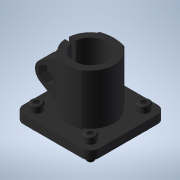
# Autodesk Inventor part: BZA-GP
Saved by Autodesk Inventor 2021 (Build 250183000, 183)
## iProperties
Created: 2025-06-23
Part Number: BZA-GP
Material: Generic
Catalog Web Link: www.cadenas.de
Description: Stands-Accessories
Vendor: RNA
Document SubType Name: Modeling
Designer: psAdmin
Manufacturer: RNA
Mass: 155.079 g
Surface Area: 462.762 cm^2
Volume: 155.079 cm^3
Density: 1 g/cm^3
Appearance: PSOLRGB-175-175-175
Category: PARTsolutions
Company: RNA
Title: BZA-GP
Author: Cadenas PARTsolutions
Comments: Accessories
PSOL_IDENT_0: {$CADENAS_DATA/23d-libs/rna/bunker/zubehoer/parts/bza_grund_110.prj},152 {VTYP=3D},{NB=BZA-GP},{LINA=
PSOL_IDENT_1: BZA-GP},{NN=Stands},{DATE=06.06.2017 07:14:33},{GEOMDATE=27.04.2017 12:08:00},{VERSION=},{LINEID=10}
PSOL_IDENT_2: ,{WBVAR=},{WBNUMERIC=}  {NB=BZA-GP},{LINA=BZA-GP},{KT=DUMMY},{IDNR=BZA-GP}
NB: BZA-GP
NN: Stands
NT: Accessories
NBSYN: $IDNR.
LINA: BZA-GP
CATALOG: Rhein-Nadel-Automation
IDNR: BZA-GP
SUPPLIER: RNA
ARTICLENO: BZA-GP
BOMINFO: BZA-GP
CREATOR: CADENAS GmbH
Autodesk Inventor part; units mm, degrees
ref_plane "YZ Plane" through (0, 0, 0) normal (1, 0, 0) x (0, 1, 0)
ref_plane "XZ Plane" through (0, 0, 0) normal (0, 1, 0) x (-1, 0, 0)
ref_plane "XY Plane" through (0, 0, 0) normal (0, 0, 1) x (1, 0, 0)
sketch "Sketch_1" plane through (0, 0, 0) normal (0, 1, 0) x (-1, 0, 0)
  line L0 (45, 2.5) -> (45, 35)
  arc A0 (45, 35) -> (35, 45) centre (35, 35) ccw
  line L1 (35, 45) -> (-35, 45)
  arc A1 (-35, 45) -> (-45, 35) centre (-35, 35) ccw
  line L2 (-45, 35) -> (-45, -35)
  arc A2 (-45, -35) -> (-35, -45) centre (-35, -35) ccw
  line L3 (-35, -45) -> (35, -45)
  arc A3 (35, -45) -> (45, -35) centre (35, -35) ccw
  line L4 (45, -35) -> (45, -2.5)
  line L5 (45, -2.5) -> (0, -2.5)
  line L6 (0, -2.5) -> (0, 2.5)
  line L7 (0, 2.5) -> (45, 2.5)
  arc A4 (-26.9948, -33.0052) -> (-33.0052, -26.9948) centre (-30, -30) ccw
  line L8 (-33.0052, -26.9948) -> (-35.0052, -28.9948)
  arc A5 (-35.0052, -28.9948) -> (-28.9948, -35.0052) centre (-32, -32) ccw
  line L9 (-28.9948, -35.0052) -> (-26.9948, -33.0052)
  arc A6 (-33.0052, 26.9948) -> (-26.9948, 33.0052) centre (-30, 30) ccw
  line L10 (-26.9948, 33.0052) -> (-28.9948, 35.0052)
  arc A7 (-28.9948, 35.0052) -> (-35.0052, 28.9948) centre (-32, 32) ccw
  line L11 (-35.0052, 28.9948) -> (-33.0052, 26.9948)
  arc A8 (28.9948, -35.0052) -> (35.0052, -28.9948) centre (32, -32) ccw
  line L12 (35.0052, -28.9948) -> (33.0052, -26.9948)
  arc A9 (33.0052, -26.9948) -> (26.9948, -33.0052) centre (30, -30) ccw
  line L13 (26.9948, -33.0052) -> (28.9948, -35.0052)
  arc A10 (35.0052, 28.9948) -> (28.9948, 35.0052) centre (32, 32) ccw
  line L14 (28.9948, 35.0052) -> (26.9948, 33.0052)
  arc A11 (26.9948, 33.0052) -> (33.0052, 26.9948) centre (30, 30) ccw
  line L15 (33.0052, 26.9948) -> (35.0052, 28.9948)
  constraints: 32 end point, 24 point on circle, 12 centre point
extrude "Extrusion1" add sketch "Sketch_1" along normal blind 10
sketch "Sketch_2" plane through (0, 10, 0) normal (0, 1, 0) x (1, 0, 0)
  arc A0 (-27.8882, -2.5) -> (-15, -23.6432) centre (0, 0) ccw
  line L0 (-15, -23.6432) -> (-15, -25.4856)
  arc A1 (-15, -25.4856) -> (15, -25.4856) centre (0, 18) ccw
  line L1 (15, -25.4856) -> (15, -23.6432)
  arc A2 (15, -23.6432) -> (15, 23.6432) centre (0, 0) ccw
  line L2 (15, 23.6432) -> (15, 25.4856)
  arc A3 (15, 25.4856) -> (-15, 25.4856) centre (0, -18) ccw
  line L3 (-15, 25.4856) -> (-15, 23.6432)
  arc A4 (-15, 23.6432) -> (-27.8882, 2.5) centre (0, 0) ccw
  line L4 (-27.8882, 2.5) -> (0, 2.5)
  line L5 (0, 2.5) -> (0, -2.5)
  line L6 (0, -2.5) -> (-27.8882, -2.5)
  constraints: 14 end point, 10 point on circle, 5 centre point
extrude "Extrusion2" add sketch "Sketch_2" along normal blind 60
sketch "Sketch_3" plane through (0, 0, 0) normal (1, 0, 0) x (0, 1, 0)
  line L0 (40, -36.5) -> (40, -26.5)
  line L1 (40, -26.5) -> (47.5, -26.5)
  line L2 (47.5, -26.5) -> (47.5, -36.5)
  line L3 (47.5, -36.5) -> (40, -36.5)
  line L4 (40, -36.5) -> (40, -26.5)
  constraints: 10 end point
revolve "Revolution1" cut sketch "Sketch_3" angle 360 about axis through (0, 40, -36.5) along (0, 0, -1)
sketch "Sketch_4" plane through (0, 0, 2.5) normal (0, 0, 1) x (1, 0, 0)
  arc A0 (-39.6142, 51.1916) -> (-39.6142, 28.8084) centre (-33, 40) ccw
  line L0 (-39.6142, 28.8084) -> (-19.1, 16.6845)
  line L1 (-19.1, 16.6845) -> (-19.1, 63.3155)
  line L2 (-19.1, 63.3155) -> (-39.6142, 51.1916)
  constraints: 6 end point, 2 point on circle, 1 centre point
extrude "Extrusion3" add sketch "Sketch_4" along normal blind 17.5
sketch "Sketch_5" plane through (0, 0, -2.5) normal (0, 0, 1) x (1, 0, 0)
  arc A0 (-39.6142, 51.1916) -> (-39.6142, 28.8084) centre (-33, 40) ccw
  line L0 (-39.6142, 28.8084) -> (-19.1, 16.6845)
  line L1 (-19.1, 16.6845) -> (-19.1, 63.3155)
  line L2 (-19.1, 63.3155) -> (-39.6142, 51.1916)
  constraints: 6 end point, 2 point on circle, 1 centre point
extrude "Extrusion4" add sketch "Sketch_5" against normal blind 17.5
sketch "Sketch_6" plane through (0, 0, 0) normal (0, 1, 0) x (-1, 0, 0)
  circle A0 centre (0, 0) radius 20.085
  constraints: 1 centre point
extrude "Extrusion5" cut sketch "Sketch_6" along normal blind 70
sketch "Sketch_7" plane through (0, 0, 20) normal (0, 0, 1) x (1, 0, 0)
  line L0 (-41.5, 35.0925) -> (-33, 30.185)
  line L1 (-33, 30.185) -> (-24.5, 35.0925)
  line L2 (-24.5, 35.0925) -> (-24.5, 44.9075)
  line L3 (-24.5, 44.9075) -> (-33, 49.815)
  line L4 (-33, 49.815) -> (-41.5, 44.9075)
  line L5 (-41.5, 44.9075) -> (-41.5, 35.0925)
  constraints: 12 end point
extrude "Extrusion6" cut sketch "Sketch_7" against normal blind 10
sketch "Sketch_8" plane through (0, 0, -20) normal (0, 0, 1) x (1, 0, 0)
  line L0 (-41.5, 35.0925) -> (-33, 30.185)
  line L1 (-33, 30.185) -> (-24.5, 35.0925)
  line L2 (-24.5, 35.0925) -> (-24.5, 44.9075)
  line L3 (-24.5, 44.9075) -> (-33, 49.815)
  line L4 (-33, 49.815) -> (-41.5, 44.9075)
  line L5 (-41.5, 44.9075) -> (-41.5, 35.0925)
  constraints: 12 end point
extrude "Extrusion7" cut sketch "Sketch_8" along normal blind 10
sketch "Sketch_10" plane through (0, 0, 0) normal (0, 0, 1) x (1, 0, 0)
  circle A0 centre (-33, 40) radius 5.25
  constraints: 1 centre point
extrude "Extrusion8" cut sketch "Sketch_10" along normal mid plane 60
sketch "Sketch_12" plane through (0, 0, 32) normal (0, 0, 1) x (1, 0, 0)
  line L0 (32, -10) -> (32, 18)
  line L1 (32, 18) -> (37.7, 18)
  line L2 (37.7, 18) -> (38.5, 17.2)
  line L3 (38.5, 17.2) -> (38.5, 10.34)
  line L4 (38.5, 10.34) -> (38.16, 10)
  line L5 (38.16, 10) -> (36.8083, 10)
  arc A0 (36.8083, 10) -> (36.4619, 9.8) centre (36.8083, 9.6) ccw
  line L6 (36.4619, 9.8) -> (36.0536, 9.0928)
  arc A1 (36.0536, 9.0928) -> (36, 8.8928) centre (36.4, 8.8928) ccw
  line L7 (36, 8.8928) -> (36, -9.233)
  line L8 (36, -9.233) -> (35.233, -10)
  line L9 (35.233, -10) -> (32, -10)
  line L10 (32, -10) -> (32, 18)
  constraints: 22 end point, 4 point on circle, 2 centre point
revolve "Revolution2" add sketch "Sketch_12" angle 360 about axis through (32, -10, 32) along (0, -1, 0)
thread "Thread1" size "M8x1.25" class "6g" standard "ISO Metric profile" length 17.233
sketch "Sketch_13" plane through (32, 18, 32) normal (0, 1, 0) x (1, 0, 0)
  line L0 (-3, -1.7321) -> (0, -3.4641)
  line L1 (0, -3.4641) -> (3, -1.7321)
  line L2 (3, -1.7321) -> (3, 1.7321)
  line L3 (3, 1.7321) -> (0, 3.4641)
  line L4 (0, 3.4641) -> (-3, 1.7321)
  line L5 (-3, 1.7321) -> (-3, -1.7321)
  constraints: 12 end point
extrude "Extrusion9" cut sketch "Sketch_13" against normal blind 4
sketch "Sketch_14" plane through (0, 0, 32) normal (0, 0, 1) x (1, 0, 0)
  line L0 (-32, -10) -> (-32, 18)
  line L1 (-32, 18) -> (-26.3, 18)
  line L2 (-26.3, 18) -> (-25.5, 17.2)
  line L3 (-25.5, 17.2) -> (-25.5, 10.34)
  line L4 (-25.5, 10.34) -> (-25.84, 10)
  line L5 (-25.84, 10) -> (-27.1917, 10)
  arc A0 (-27.1917, 10) -> (-27.5381, 9.8) centre (-27.1917, 9.6) ccw
  line L6 (-27.5381, 9.8) -> (-27.9464, 9.0928)
  arc A1 (-27.9464, 9.0928) -> (-28, 8.8928) centre (-27.6, 8.8928) ccw
  line L7 (-28, 8.8928) -> (-28, -9.233)
  line L8 (-28, -9.233) -> (-28.767, -10)
  line L9 (-28.767, -10) -> (-32, -10)
  line L10 (-32, -10) -> (-32, 18)
  constraints: 22 end point, 4 point on circle, 2 centre point
revolve "Revolution3" add sketch "Sketch_14" angle 360 about axis through (-32, -10, 32) along (0, -1, 0)
thread "Thread2" size "M8x1.25" class "6g" standard "ISO Metric profile" length 17.233
sketch "Sketch_15" plane through (-32, 18, 32) normal (0, 1, 0) x (1, 0, 0)
  line L0 (-3, -1.7321) -> (0, -3.4641)
  line L1 (0, -3.4641) -> (3, -1.7321)
  line L2 (3, -1.7321) -> (3, 1.7321)
  line L3 (3, 1.7321) -> (0, 3.4641)
  line L4 (0, 3.4641) -> (-3, 1.7321)
  line L5 (-3, 1.7321) -> (-3, -1.7321)
  constraints: 12 end point
extrude "Extrusion10" cut sketch "Sketch_15" against normal blind 4
sketch "Sketch_16" plane through (0, 0, -32) normal (0, 0, 1) x (1, 0, 0)
  line L0 (32, -10) -> (32, 18)
  line L1 (32, 18) -> (37.7, 18)
  line L2 (37.7, 18) -> (38.5, 17.2)
  line L3 (38.5, 17.2) -> (38.5, 10.34)
  line L4 (38.5, 10.34) -> (38.16, 10)
  line L5 (38.16, 10) -> (36.8083, 10)
  arc A0 (36.8083, 10) -> (36.4619, 9.8) centre (36.8083, 9.6) ccw
  line L6 (36.4619, 9.8) -> (36.0536, 9.0928)
  arc A1 (36.0536, 9.0928) -> (36, 8.8928) centre (36.4, 8.8928) ccw
  line L7 (36, 8.8928) -> (36, -9.233)
  line L8 (36, -9.233) -> (35.233, -10)
  line L9 (35.233, -10) -> (32, -10)
  line L10 (32, -10) -> (32, 18)
  constraints: 22 end point, 4 point on circle, 2 centre point
revolve "Revolution4" add sketch "Sketch_16" angle 360 about axis through (32, -10, -32) along (0, -1, 0)
thread "Thread3" size "M8x1.25" class "6g" standard "ISO Metric profile" length 17.233
sketch "Sketch_17" plane through (0, 0, -32) normal (0, 0, 1) x (1, 0, 0)
  line L0 (-32, -10) -> (-32, 18)
  line L1 (-32, 18) -> (-26.3, 18)
  line L2 (-26.3, 18) -> (-25.5, 17.2)
  line L3 (-25.5, 17.2) -> (-25.5, 10.34)
  line L4 (-25.5, 10.34) -> (-25.84, 10)
  line L5 (-25.84, 10) -> (-27.1917, 10)
  arc A0 (-27.1917, 10) -> (-27.5381, 9.8) centre (-27.1917, 9.6) ccw
  line L6 (-27.5381, 9.8) -> (-27.9464, 9.0928)
  arc A1 (-27.9464, 9.0928) -> (-28, 8.8928) centre (-27.6, 8.8928) ccw
  line L7 (-28, 8.8928) -> (-28, -9.233)
  line L8 (-28, -9.233) -> (-28.767, -10)
  line L9 (-28.767, -10) -> (-32, -10)
  line L10 (-32, -10) -> (-32, 18)
  constraints: 22 end point, 4 point on circle, 2 centre point
revolve "Revolution5" add sketch "Sketch_17" angle 360 about axis through (-32, -10, -32) along (0, -1, 0)
thread "Thread4" size "M8x1.25" class "6g" standard "ISO Metric profile" length 17.233
sketch "Sketch_18" plane through (32, 18, -32) normal (0, 1, 0) x (1, 0, 0)
  line L0 (-3, -1.7321) -> (0, -3.4641)
  line L1 (0, -3.4641) -> (3, -1.7321)
  line L2 (3, -1.7321) -> (3, 1.7321)
  line L3 (3, 1.7321) -> (0, 3.4641)
  line L4 (0, 3.4641) -> (-3, 1.7321)
  line L5 (-3, 1.7321) -> (-3, -1.7321)
  constraints: 12 end point
extrude "Extrusion11" cut sketch "Sketch_18" against normal blind 4
sketch "Sketch_19" plane through (-32, 18, -32) normal (0, 1, 0) x (1, 0, 0)
  line L0 (-3, -1.7321) -> (0, -3.4641)
  line L1 (0, -3.4641) -> (3, -1.7321)
  line L2 (3, -1.7321) -> (3, 1.7321)
  line L3 (3, 1.7321) -> (0, 3.4641)
  line L4 (0, 3.4641) -> (-3, 1.7321)
  line L5 (-3, 1.7321) -> (-3, -1.7321)
  constraints: 12 end point
extrude "Extrusion12" cut sketch "Sketch_19" against normal blind 4
ref_plane "DUMMY_XY" through (0, 0, 0) normal (0, 1, 0) x (1, 0, 0)
ref_plane "DUMMY_YZ" through (0, 0, 0) normal (1, 0, 0) x (0, 0, -1)
ref_plane "DUMMY_ZX" through (0, 0, 0) normal (0, 0, -1) x (0, 1, 0)
ref_plane "PROFIL_XY" through (0, 0, 0) normal (0, -1, 0) x (1, 0, 0)
ref_plane "PROFIL_YZ" through (0, 0, 0) normal (1, 0, 0) x (0, 0, 1)
ref_plane "PROFIL_ZX" through (0, 0, 0) normal (0, 0, 1) x (0, -1, 0)
ref_plane "SCHRAUBE_XY" through (-33, 40, -10) normal (0, 0, 1) x (1, 0, 0)
ref_plane "SCHRAUBE_YZ" through (-33, 40, -10) normal (1, 0, 0) x (0, 1, 0)
ref_plane "SCHRAUBE_ZX" through (-33, 40, -10) normal (0, 1, 0) x (0, 0, 1)
body "Solid1"
